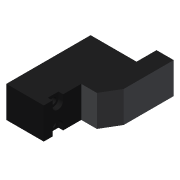
# Autodesk Inventor part: Valve_Outside
Saved by Autodesk Inventor 2016 (Build 200138000, 138)
## iProperties
Created: 2011-10-12
Part Number: Valve_Outside
Document SubType Name: Modeling
Designer: Neef
Density: 1 g/cm^3
Material: Generic
Appearance: Magenta
Author: Neef
Autodesk Inventor part; units mm, degrees
note: some values were not read from the file. Chosen so that the rebuilt part matches the saved one: direction of "Bohrung1".
ref_plane "YZ Plane" through (0, 0, 0) normal (1, 0, 0) x (0, 1, 0)
ref_plane "XZ Plane" through (0, 0, 0) normal (0, 1, 0) x (-1, 0, 0)
ref_plane "XY Plane" through (0, 0, 0) normal (0, 0, 1) x (1, 0, 0)
sketch "Skizze1" plane through (0, 0, 0) normal (0, 0, 1) x (1, 0, 0)
  line L0 (0, 40.08) -> (0, -6.68) projected
  line L1 (-4.04, 0) -> (24.24, 0) projected
  line L2 (0, 0) -> (12, 0)
  line L3 (12, 0) -> (12, 12)
  line L4 (14.7, 27) -> (0, 27)
  line L5 (0, 27) -> (0, 0)
  line L6 (14.7, 27) -> (14.7, 33.4)
  line L7 (14.7, 33.4) -> (20.2, 33.4)
  line L8 (20.2, 33.4) -> (20.2, 17.4)
  line L9 (20.2, 17.4) -> (17, 12)
  line L10 (17, 12) -> (12, 12)
  dimension "d0" = 5.5
  dimension "d1" = 14.7
  dimension "d3" = 12
  dimension "d4" = 27
  dimension "d5" = 12
  dimension "d6" = 5
  dimension "d7" = 6.4
  dimension "d8" = 16
  constraints: 18 end point, 4 parallel, 3 perpendicular, 2 point on line, 1 horizontal
  measures "d0" distance of L6.end L7.end
  measures "d1" distance of L4.start L4.end
  measures "d3" distance between parallel lines of L0 L3
  measures "d4" distance between parallel lines of L1 L4
  measures "d5" distance of L2.end L3.end
  measures "d6" distance of L9.end L3.end
  measures "d7" distance of L4.start L6.end
  measures "d8" distance of L7.end L8.end
extrude "Extrusion1" add sketch "Skizze1" along normal mid plane 10
hole "Bohrung1" at (12, 4.5, 3.25) direction (-1, 0, 0) diameter 2 end up to surface counterbore diameter 3.4 counterbore depth 1.5
sketch "Skizze2" plane through (12, 0, -5) normal (1, 0, 0) x (0, 0, -1)
  circle A0 centre (-8.25, 4.5) radius 1.7 projected
  line L0 (-10, 0) -> (-10, 27) projected
  line L1 (-10, 2.8) -> (-8.25, 2.8)
  line L2 (-8.25, 2.8) -> (-8.25, 6.2)
  line L3 (-8.25, 6.2) -> (-10, 6.2)
  line L4 (-10, 6.2) -> (-10, 2.8)
  point P0 (-10, 5.3874)
  point P1 (-10, 3.6126)
  constraints: 8 end point, 3 horizontal, 2 parallel, 1 perpendicular, 1 point on line, 1 other
extrude "Extrusion2" cut sketch "Skizze2" against normal up to surface (1.5 mm away) contours L2 A0 | A0 L1 L0 L3 picked at (-8.7614, 4.0923)
mirror "Spiegeln1" about plane through (0, 0, 0) normal (0, 0, 1) of "Bohrung1", "Extrusion2"
sketch "Skizze3" plane through (0, 0, 5) normal (-1, 0, 0) x (0, 0, 1)
  line L0 (0, 0) -> (0, 27) projected
  line L1 (0, 0) -> (-10, 0) projected
  circle A0 centre (-1.75, 4.5) radius 1 projected
  point P0 (-5, 2.8)
  point P1 (-5, 5.3)
  point P2 (-5, 7.8)
  dimension "d22" = 2.5
  dimension "d23" = 2.5
  dimension "d24" = 2.8
  dimension "d25" = 7.8
  dimension "d26" = 5
  dimension "d27" = 5.3
  dimension "d35" = 0.8
  measures "d22" distance of point (-5, 5.3) point (-5, 2.8)
  measures "d23" distance of point (-5, 7.8) point (-5, 5.3)
  measures "d24" distance from line of point (-5, 2.8) L1
  measures "d25" distance from line of point (-5, 7.8) L1
  measures "d26" distance from line of point (-5, 7.8) L0
  measures "d27" distance from line of point (-5, 5.3) L1
  measures "d35" vertical distance of point (-5, 5.3) A0.centre
hole "Bohrung2" at (0, 2.8, 0) at (0, 5.3, 0) at (0, 7.8, 0) direction (1, 0, 0) diameter 1.5 depth 8 tip angle 118
equation "\"d23\" = d22"
